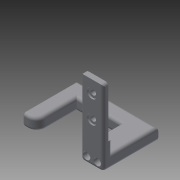
# Autodesk Inventor part: bed-hook
Saved by Autodesk Inventor 2014 (Build 180170000, 170)
## iProperties
Created: 2017-07-21
Part Number: bed-hook
Material: 一般
Document SubType Name: Modeling
Designer: hide
Density: 1 g/cm^3
Appearance: 既定
Author: hide
Autodesk Inventor part; units mm, degrees
ref_plane "YZ Plane" through (0, 0, 0) normal (1, 0, 0) x (0, 1, 0)
ref_plane "XZ Plane" through (0, 0, 0) normal (0, 1, 0) x (-1, 0, 0)
ref_plane "XY Plane" through (0, 0, 0) normal (0, 0, 1) x (1, 0, 0)
sketch "スケッチ1" plane through (0, 0, 0) normal (0, 1, 0) x (-1, 0, 0)
  line L0 (0, 0) -> (15, 0)
  line L1 (15, 0) -> (15, -50)
  line L2 (15, -50) -> (0, -50)
  line L3 (0, -50) -> (0, 0)
  circle A0 centre (7.5, -8) radius 1.75
  circle A1 centre (7.5, -23) radius 1.75
  dimension "d0" = 15
  dimension "d1" = 50
  dimension "d2" = 15
  dimension "d3" = 3.5
  dimension "d4" = 3.5
  dimension "d5" = 0
  dimension "d6" = 7.5
  dimension "d7" = 8
  constraints: 8 end point, 2 centre point, 2 parallel, 1 horizontal, 1 perpendicular
  measures "d0" distance of L0.start L0.end
  measures "d1" distance of L2.end L0.start
  measures "d2" distance of A1.centre A0.centre
  measures "d3" diameter of A0
  measures "d4" diameter of A1
  measures "d5" horizontal distance of A1.centre A0.centre
  measures "d6" distance from line of L3 A0.centre
  measures "d7" distance from line of L0 A0.centre
extrude "押し出し1" add sketch "スケッチ1" along normal blind 6
sketch "スケッチ2" plane through (0, 6, 0) normal (0, 1, 0) x (1, 0, 0)
  line L0 (0, 0) -> (0, 50) projected
  line L1 (0, 50) -> (-15, 50) projected
  line L2 (-15, 50) -> (0, 50)
  line L3 (0, 50) -> (0, 42)
  line L4 (0, 42) -> (-15, 42)
  line L5 (-15, 42) -> (-15, 50)
  dimension "d10" = 8
  constraints: 8 end point, 2 parallel, 1 horizontal, 1 perpendicular, 1 point on line
  measures "d10" distance of L4.end L1.end
extrude "押し出し2" add sketch "スケッチ2" along normal blind 20.5
sketch "スケッチ3" plane through (0, 26.5, 0) normal (0, 1, 0) x (1, 0, 0)
  line L0 (-15, 50) -> (-15, 42) projected
  line L1 (0, 42) -> (-44, 42)
  line L2 (-44, 42) -> (-44, 50)
  line L3 (-44, 50) -> (0, 50)
  line L4 (0, 50) -> (0, 42)
  point P0 (0, 0)
  dimension "d13" = 29
  dimension "d14" = 8
  constraints: 8 end point, 2 parallel, 1 horizontal, 1 perpendicular
  measures "d13" distance between parallel lines of L0 L2
  measures "d14" distance of L1.end L2.end
extrude "押し出し3" add sketch "スケッチ3" along normal blind 10
sketch "スケッチ4" plane through (-44, 26.5, -50) normal (-1, 0, 0) x (0, 0, 1)
  line L0 (50, -26.5) -> (0, -26.5) projected
  line L1 (50, -26.5) -> (50, -20.5) projected
  line L2 (8, -20.5) -> (50, -20.5) projected
  line L3 (8, -20.5) -> (8, 0) projected
  line L4 (0, 0) -> (8, 0) projected
  line L5 (0, -26.5) -> (0, 0) projected
  line L6 (8, 10) -> (0, 10)
  line L7 (0, 10) -> (0, -26.5)
  line L8 (0, -26.5) -> (8, -26.5)
  line L9 (8, -26.5) -> (8, 10)
  point P0 (50, -26.5)
  constraints: 8 end point, 2 parallel, 1 horizontal, 1 perpendicular
extrude "押し出し4" add sketch "スケッチ4" along normal blind 10 contours L0 L5 L4 L3 L9 | L7 L6 L9 L4
fillet "フィレット1" radius 6 1 edges at (-44, 0, -46)
fillet "フィレット2" radius 2 23 edges at (-44, 16.25, -42) (-52, 0, -42) (-29.5, 26.5, -42) (-15, 16.25, -42) (0, 18.25, -50) (-27, 36.5, -50) (-54, 18.25, -42) (-54, 18.25, -50) (-54, 0, -46) (-44, 16.25, -50) (-52, 0, -50) (-15, 6, -21) (-7.5, 6, 0) (0, 6, -21) (0, 3, 0) (-15, 13.25, -50) (0, 21.25, -42) (-27, 36.5, -42) (-15, 3, 0) (-29.5, 26.5, -50) (-7.5, 0, -50) (-15, 0, -25) (0, 0, -25)
sketch "スケッチ5" plane through (0, 6, 0) normal (0, 1, 0) x (1, 0, 0)
  circle A0 centre (-7.5, 8) radius 1.75 projected
  circle A1 centre (-7.5, 23) radius 1.75 projected
  line L0 (-15, 44) -> (-15, 2) projected
  line L1 (-15, 2) -> (-13, 2) projected
  line L2 (-13, 2) -> (-13, 42) projected
  arc A2 (-15, 44) -> (-13, 42) centre (-13, 44) ccw projected
  line L3 (-2, 42) -> (-2, 2) projected
  line L4 (-2, 2) -> (0, 2) projected
  line L5 (0, 2) -> (0, 44) projected
  arc A3 (-2, 42) -> (0, 44) centre (-2, 44) ccw projected
  line L6 (-2, 0) -> (-2, 2) projected
  line L7 (-2, 2) -> (-13, 2) projected
  line L8 (-13, 2) -> (-13, 0) projected
  line L9 (-13, 0) -> (-2, 0) projected
  line L10 (-15, 33.6) -> (0, 33.6)
  line L11 (0, 33.6) -> (0, -0.8351)
  line L12 (0, -0.8351) -> (-15, -0.8351)
  line L13 (-15, -0.8351) -> (-15, 33.6)
  point P0 (0, 0)
  dimension "d21" = 10.6
  constraints: 8 end point, 2 parallel, 1 horizontal, 1 perpendicular, 1 point on line
  measures "d21" distance from line of L10 A1.centre
extrude "押し出し5" cut sketch "スケッチ5" against normal blind 2.5 contours A0 | A1 | L10 L2 L1 L0 | L1 L8 L9 L6 L4 L11 L12 L13 | L10 L3 L7 L2 | L7 L6 L9 L8 | L10 L5 L4 L3
sketch "スケッチ6" plane through (0, 0, 0) normal (0, -1, 0) x (1, 0, 0)
  circle A0 centre (-10.9574, -45.6442) radius 1.4
  circle A1 centre (-3.9574, -45.6442) radius 1.4
  point P0 (0, 0)
  dimension "d24" = 2.8
  dimension "d25" = 2.8
  dimension "d26" = 0
  dimension "d27" = 7
  constraints: 2 centre point
  measures "d24" diameter of A0
  measures "d25" diameter of A1
  measures "d26" vertical distance of A1.centre A0.centre
  measures "d27" distance of A1.centre A0.centre
extrude "押し出し6" cut sketch "スケッチ6" against normal blind 15
sketch "スケッチ7" plane through (0, 0, 0) normal (0, -1, 0) x (1, 0, 0)
  circle A0 centre (-10.9574, -45.6442) radius 1.4 projected
  circle A1 centre (-3.9574, -45.6442) radius 1.4 projected
  circle A2 centre (-10.9574, -45.6442) radius 2.4
  circle A3 centre (-3.9574, -45.6442) radius 2.4
  point P0 (0, 0)
  dimension "d30" = 1
  dimension "d31" = 1
  constraints: 2 centre point, 2 coincident
  measures "d30" radial gap between concentric circles of A2 A0
  measures "d31" radial gap between concentric circles of A3 A1
extrude "押し出し7" cut sketch "スケッチ7" against normal blind 3
fillet "フィレット3" radius 1 2 edges at (-13.3574, 3, -45.6442) (-6.3574, 3, -45.6442)
sketch "スケッチ8" plane through (0, 0, 0) normal (0, -1, 0) x (1, 0, 0)
  circle A0 centre (-7.5, -23) radius 1.75 projected
  circle A1 centre (-7.5, -8) radius 1.75 projected
  circle A2 centre (-7.5, -8) radius 3.25
  circle A3 centre (-7.5, -23) radius 3.25
  point P0 (0, 0)
  dimension "d35" = 1.5
  dimension "d36" = 1.5
  constraints: 2 centre point, 2 coincident
  measures "d35" radial gap between concentric circles of A2 A1
  measures "d36" radial gap between concentric circles of A3 A0
extrude "押し出し8" cut sketch "スケッチ8" against normal blind 1
equation "\"d4\" = d3"
equation "\"d6\" = 0.5 * d0"
equation "\"d25\" = d24"
equation "\"d31\" = d30"
equation "\"d36\" = d35"
